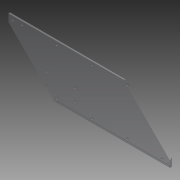
# Autodesk Inventor part: Hopper Right
Saved by Autodesk Inventor 2014 SP1 (Build 180222100, 222)
## iProperties
Created: 2013-12-16
Part Number: Hopper Right
Material: Polycarbonate, Clear
Document SubType Name: Modeling
Designer: Moses
Mass: 135.195 g
Surface Area: 743.202 cm^2
Volume: 112.662 cm^3
Density: 1.2 g/cm^3
Appearance: Polycarbonate - Clear
Author: Moses
Autodesk Inventor part; units mm, degrees
ref_plane "YZ Plane" through (0, 0, 0) normal (1, 0, 0) x (0, 1, 0)
ref_plane "XZ Plane" through (0, 0, 0) normal (0, 1, 0) x (-1, 0, 0)
ref_plane "XY Plane" through (0, 0, 0) normal (0, 0, 1) x (1, 0, 0)
sketch "Sketch1" plane through (0, 0, 0) normal (0, 0, 1) x (1, 0, 0)
  line L0 (330.2, 0) -> (330.2, 107.8942)
  line L1 (330.2, 107.8942) -> (0, 107.8942)
  line L2 (0, 107.8942) -> (0, 0)
  line L3 (0, 0) -> (330.2, 0)
  circle A0 centre (97.6313, 100.3536) radius 1.5875 projected
  circle A1 centre (240.5063, 100.3536) radius 1.5875 projected
  circle A2 centre (311.9438, 100.3536) radius 1.5875 projected
  circle A3 centre (169.0688, 100.3536) radius 1.5875 projected
  circle A4 centre (26.1938, 100.3536) radius 1.5875 projected
  line L4 (321.4688, 107.8942) -> (321.4688, 92.8129) construction
  line L5 (321.4688, 107.8942) -> (16.6688, 107.8942) construction
  line L6 (16.6688, 92.8129) -> (16.6688, 107.8942) construction
  line L7 (321.4688, 92.8129) -> (16.6688, 92.8129) construction
  circle A5 centre (97.6313, 5.2784) radius 1.5875 projected
  circle A6 centre (240.5063, 5.2784) radius 1.5875 projected
  circle A7 centre (311.9438, 5.2784) radius 1.5875 projected
  circle A8 centre (169.0688, 5.2784) radius 1.5875 projected
  circle A9 centre (26.1938, 5.2784) radius 1.5875 projected
  line L8 (321.4688, 12.819) -> (321.4688, -2.2623) construction
  line L9 (321.4688, 12.819) -> (16.6688, 12.819) construction
  line L10 (16.6688, -2.2623) -> (16.6688, 12.819) construction
  line L11 (321.4688, -2.2623) -> (16.6688, -2.2623) construction
  circle A10 centre (19.8438, 18.3592) radius 1.5875 projected
  circle A11 centre (76.9938, 18.3592) radius 1.5875 projected
  circle A12 centre (134.1438, 18.3592) radius 1.5875 projected
  circle A13 centre (19.8438, 43.7592) radius 1.5875 projected
  circle A14 centre (76.9938, 43.7592) radius 1.5875 projected
  circle A15 centre (134.1438, 43.7592) radius 1.5875 projected
  line L12 (143.6688, 53.2842) -> (143.6688, -124.5158) construction
  line L13 (16.6688, 53.2842) -> (143.6688, 53.2842) construction
  line L14 (16.6688, 2.4842) -> (16.6688, 53.2842) construction
  line L15 (143.6688, -124.5158) -> (-72.2312, -124.5158) construction
  circle A16 centre (7.5406, 99.1629) radius 1.5875 projected
  circle A17 centre (7.5406, 16.6129) radius 1.5875 projected
  line L16 (0, 108.6879) -> (15.0813, 108.6879) construction
  line L17 (0, 108.6879) -> (0, 7.0879) construction
  line L18 (15.0813, 7.0879) -> (0, 7.0879) construction
  line L19 (15.0813, 108.6879) -> (15.0813, 7.0879) construction
  line L20 (3.9688, 2.4842) -> (16.6688, 2.4842) projected
  line L21 (-72.2312, -124.5158) -> (3.9688, 2.4842) projected
  dimension "d0" = 330.2
  dimension "d1" = 107.8942
  constraints: 8 end point, 2 perpendicular, 1 coincident, 1 horizontal, 1 vertical
  measures "d0" distance of L0.end L1.end
  measures "d1" distance of L1.end L2.end
extrude "Extrusion1" add sketch "Sketch1" along normal blind 3.175
body "Solid1"
